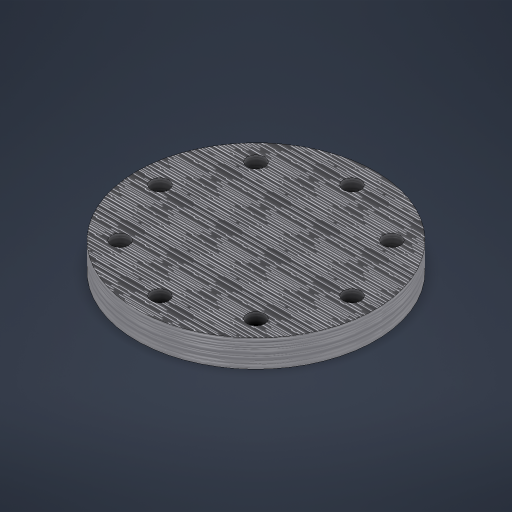
# Autodesk Inventor part: BearingSpacerPlate
Saved by Autodesk Inventor 2024 (Build 280153000, 153)
## iProperties
Created: 2024-01-05
Part Number: BearingSpacerPlate
Material: Generic
Document SubType Name: Modeling
Designer: avsar
Density: 1 g/cm^3
Appearance: Machined 03
Author: avsar
Autodesk Inventor part; units mm, degrees
ref_plane "YZ Plane" through (0, 0, 0) normal (1, 0, 0) x (0, 1, 0)
ref_plane "XZ Plane" through (0, 0, 0) normal (0, 1, 0) x (-1, 0, 0)
ref_plane "XY Plane" through (0, 0, 0) normal (0, 0, 1) x (1, 0, 0)
sketch "Sketch1" plane through (0, 0, 0) normal (0, 1, 0) x (-1, 0, 0)
  circle A0 centre (0, 0) radius 28
  dimension "d0" = 56
  constraints: 1 centre point, 1 coincident
  measures "d0" diameter of A0
extrude "Extrusion1" add sketch "Sketch1" along normal mid plane 6.35
sketch "Sketch2" plane through (0, 3.175, 0) normal (0, 1, 0) x (1, 0, 0)
  circle A0 centre (0, 22.5) radius 2.05
  circle A1 centre (-15.9099, 15.9099) radius 2.05
  circle A2 centre (-22.5, 0) radius 2.05
  circle A3 centre (-15.9099, -15.9099) radius 2.05
  circle A4 centre (0, -22.5) radius 2.05
  circle A5 centre (15.9099, -15.9099) radius 2.05
  circle A6 centre (22.5, 0) radius 2.05
  circle A7 centre (15.9099, 15.9099) radius 2.05
  point P0 (0, 0)
  dimension "d3" = 4.1
  dimension "d4" = 22.5
  dimension "d7" = 360
  constraints: 8 centre point, 1 vertical alignment, 17 other
  measures "d3" diameter of A0
  measures "d4" distance of point (0, 0) A0.centre
extrude "Extrusion2" cut sketch "Sketch2" against normal through all
body "Solid1"
